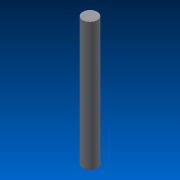
# Autodesk Inventor part: eje
Saved by Autodesk Inventor 2013 (Build 170138000, 138)
## iProperties
Created: 2013-10-20
Part Number: eje
Material: Generic
Document SubType Name: Modeling
Designer: Miguel
Density: 1 g/cm^3
Author: Miguel
Autodesk Inventor part; units mm, degrees
ref_plane "YZ Plane" through (0, 0, 0) normal (1, 0, 0) x (0, 1, 0)
ref_plane "XZ Plane" through (0, 0, 0) normal (0, 1, 0) x (-1, 0, 0)
ref_plane "XY Plane" through (0, 0, 0) normal (0, 0, 1) x (1, 0, 0)
sketch "Boceto1" plane through (0, 0, 0) normal (0, 0, 1) x (1, 0, 0)
  circle A0 centre (-0.8813, 0.6609) radius 28.5
  point P0 (0, 0)
  dimension "d0" = 57
  dimension "d0" = 57
  constraints: 1 centre point
  measures "d0" diameter of A0
extrude "Extrusión1" add sketch "Boceto1" along normal blind 500
